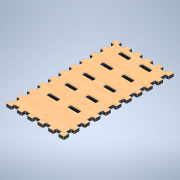
# Autodesk Inventor part: plate_top_middle
Saved by Autodesk Inventor 2021 (Build 250183000, 183)
## iProperties
Created: 2021-03-07
Part Number: plate_top_middle
Material: Holz (Kirsche)
Document SubType Name: Modeling
Designer: Tilman
Density: 0.63 g/cm^3
Appearance: Glänzend - Schwarz
Author: Tilman
Autodesk Inventor part; units mm, degrees
ref_plane "YZ Plane" through (0, 0, 0) normal (1, 0, 0) x (0, 1, 0)
ref_plane "XZ Plane" through (0, 0, 0) normal (0, 1, 0) x (-1, 0, 0)
ref_plane "XY Plane" through (0, 0, 0) normal (0, 0, 1) x (1, 0, 0)
sketch "Skizze1" plane through (0, 0, 0) normal (0, 1, 0) x (-1, 0, 0)
  line L0 (-12.5, -26) -> (-22.5, -26)
  line L1 (-22.5, -26) -> (-22.5, -29)
  line L2 (-22.5, -29) -> (-12.5, -29)
  line L3 (-12.5, -29) -> (-12.5, -26)
  line L4 (-32.5, -26) -> (-42.5, -26)
  line L5 (-42.5, -26) -> (-42.5, -29)
  line L6 (-42.5, -29) -> (-32.5, -29)
  line L7 (-32.5, -29) -> (-32.5, -26)
  line L8 (-12.5, -43) -> (-22.5, -43)
  line L9 (-22.5, -43) -> (-22.5, -46)
  line L10 (-22.5, -46) -> (-12.5, -46)
  line L11 (-12.5, -46) -> (-12.5, -43)
  line L12 (-32.5, -43) -> (-42.5, -43)
  line L13 (-42.5, -43) -> (-42.5, -46)
  line L14 (-42.5, -46) -> (-32.5, -46)
  line L15 (-32.5, -46) -> (-32.5, -43)
  line L16 (-12.5, -60) -> (-22.5, -60)
  line L17 (-22.5, -60) -> (-22.5, -63)
  line L18 (-22.5, -63) -> (-12.5, -63)
  line L19 (-12.5, -63) -> (-12.5, -60)
  line L20 (-32.5, -60) -> (-42.5, -60)
  line L21 (-42.5, -60) -> (-42.5, -63)
  line L22 (-42.5, -63) -> (-32.5, -63)
  line L23 (-32.5, -63) -> (-32.5, -60)
  line L24 (-12.5, -77) -> (-22.5, -77)
  line L25 (-22.5, -77) -> (-22.5, -80)
  line L26 (-22.5, -80) -> (-12.5, -80)
  line L27 (-12.5, -80) -> (-12.5, -77)
  line L28 (-32.5, -77) -> (-42.5, -77)
  line L29 (-42.5, -77) -> (-42.5, -80)
  line L30 (-42.5, -80) -> (-32.5, -80)
  line L31 (-32.5, -80) -> (-32.5, -77)
  line L32 (-12.5, -94) -> (-22.5, -94)
  line L33 (-22.5, -94) -> (-22.5, -97)
  line L34 (-22.5, -97) -> (-12.5, -97)
  line L35 (-12.5, -97) -> (-12.5, -94)
  line L36 (-32.5, -94) -> (-42.5, -94)
  line L37 (-42.5, -94) -> (-42.5, -97)
  line L38 (-42.5, -97) -> (-32.5, -97)
  line L39 (-32.5, -97) -> (-32.5, -94)
  line L40 (0, 0) -> (-5, 0)
  line L41 (-5, 0) -> (-5, -3)
  line L42 (-5, -3) -> (-10, -3)
  line L43 (-10, -3) -> (-10, 0)
  line L44 (-20, -3) -> (-20, 0)
  line L45 (-15, -3) -> (-20, -3)
  line L46 (-15, 0) -> (-15, -3)
  line L47 (-10, 0) -> (-15, 0)
  line L48 (-30, -3) -> (-30, 0)
  line L49 (-25, -3) -> (-30, -3)
  line L50 (-25, 0) -> (-25, -3)
  line L51 (-20, 0) -> (-25, 0)
  line L52 (-40, -3) -> (-40, 0)
  line L53 (-35, -3) -> (-40, -3)
  line L54 (-35, 0) -> (-35, -3)
  line L55 (-30, 0) -> (-35, 0)
  line L56 (-50, -3) -> (-50, 0)
  line L57 (-45, -3) -> (-50, -3)
  line L58 (-45, 0) -> (-45, -3)
  line L59 (-40, 0) -> (-45, 0)
  line L60 (-50, 0) -> (-55, 0)
  line L61 (-55, 0) -> (-55, -5)
  line L62 (-55, -5) -> (-52, -5)
  line L63 (-52, -5) -> (-52, -10)
  line L64 (-52, -10) -> (-55, -10)
  line L65 (-52, -15) -> (-52, -20)
  line L66 (-55, -10) -> (-55, -15)
  line L67 (-55, -15) -> (-52, -15)
  line L68 (-52, -20) -> (-55, -20)
  line L69 (-52, -25) -> (-52, -30)
  line L70 (-55, -20) -> (-55, -25)
  line L71 (-55, -25) -> (-52, -25)
  line L72 (-52, -30) -> (-55, -30)
  line L73 (-52, -35) -> (-52, -40)
  line L74 (-55, -30) -> (-55, -35)
  line L75 (-55, -35) -> (-52, -35)
  line L76 (-52, -40) -> (-55, -40)
  line L77 (-52, -45) -> (-52, -50)
  line L78 (-55, -40) -> (-55, -45)
  line L79 (-55, -45) -> (-52, -45)
  line L80 (-52, -50) -> (-55, -50)
  line L81 (-52, -55) -> (-52, -60)
  line L82 (-55, -50) -> (-55, -55)
  line L83 (-55, -55) -> (-52, -55)
  line L84 (-52, -60) -> (-55, -60)
  line L85 (-52, -65) -> (-52, -70)
  line L86 (-55, -60) -> (-55, -65)
  line L87 (-55, -65) -> (-52, -65)
  line L88 (-52, -70) -> (-55, -70)
  line L89 (-52, -75) -> (-52, -80)
  line L90 (-55, -70) -> (-55, -75)
  line L91 (-55, -75) -> (-52, -75)
  line L92 (-52, -80) -> (-55, -80)
  line L93 (-22.5, -61.5) -> (-32.5, -61.5) construction
  line L94 (-27.5, -105) -> (-27.5, 0) construction
  line L95 (-55, -80) -> (-55, -85)
  line L96 (-55, -105) -> (-50, -105)
  line L97 (-50, -105) -> (-50, -102)
  line L98 (-50, -102) -> (-45, -102)
  line L99 (-45, -102) -> (-45, -105)
  line L100 (-40, -102) -> (-35, -102)
  line L101 (-35, -102) -> (-35, -105)
  line L102 (-40, -105) -> (-40, -102)
  line L103 (-45, -105) -> (-40, -105)
  line L104 (-30, -102) -> (-25, -102)
  line L105 (-25, -102) -> (-25, -105)
  line L106 (-30, -105) -> (-30, -102)
  line L107 (-35, -105) -> (-30, -105)
  line L108 (-20, -102) -> (-15, -102)
  line L109 (-15, -102) -> (-15, -105)
  line L110 (-20, -105) -> (-20, -102)
  line L111 (-25, -105) -> (-20, -105)
  line L112 (-10, -102) -> (-5, -102)
  line L113 (-5, -102) -> (-5, -105)
  line L114 (-10, -105) -> (-10, -102)
  line L115 (-15, -105) -> (-10, -105)
  line L116 (-5, -105) -> (0, -105)
  line L117 (0, -105) -> (0, -100)
  line L118 (0, -100) -> (-3, -100)
  line L119 (-3, -100) -> (-3, -95)
  line L120 (-3, -95) -> (0, -95)
  line L121 (-3, -90) -> (-3, -85)
  line L122 (-3, -85) -> (0, -85)
  line L123 (0, -90) -> (-3, -90)
  line L124 (0, -95) -> (0, -90)
  line L125 (-3, -80) -> (-3, -75)
  line L126 (-3, -75) -> (0, -75)
  line L127 (0, -80) -> (-3, -80)
  line L128 (0, -85) -> (0, -80)
  line L129 (-3, -70) -> (-3, -65)
  line L130 (-3, -65) -> (0, -65)
  line L131 (0, -70) -> (-3, -70)
  line L132 (0, -75) -> (0, -70)
  line L133 (-3, -60) -> (-3, -55)
  line L134 (-3, -55) -> (0, -55)
  line L135 (0, -60) -> (-3, -60)
  line L136 (0, -65) -> (0, -60)
  line L137 (-3, -50) -> (-3, -45)
  line L138 (-3, -45) -> (0, -45)
  line L139 (0, -50) -> (-3, -50)
  line L140 (0, -55) -> (0, -50)
  line L141 (-3, -40) -> (-3, -35)
  line L142 (-3, -35) -> (0, -35)
  line L143 (0, -40) -> (-3, -40)
  line L144 (0, -45) -> (0, -40)
  line L145 (-3, -30) -> (-3, -25)
  line L146 (-3, -25) -> (0, -25)
  line L147 (0, -30) -> (-3, -30)
  line L148 (0, -35) -> (0, -30)
  line L149 (-52, -85) -> (-52, -90)
  line L150 (-55, -80) -> (-55, -85)
  line L151 (-55, -85) -> (-52, -85)
  line L152 (-52, -90) -> (-55, -90)
  line L153 (-3, -20) -> (-3, -15)
  line L154 (-3, -15) -> (0, -15)
  line L155 (0, -20) -> (-3, -20)
  line L156 (0, -25) -> (0, -20)
  line L157 (-52, -95) -> (-52, -100)
  line L158 (-55, -90) -> (-55, -95)
  line L159 (-55, -95) -> (-52, -95)
  line L160 (-52, -100) -> (-55, -100)
  line L161 (-3, -10) -> (-3, -5)
  line L162 (-3, -5) -> (0, -5)
  line L163 (0, -10) -> (-3, -10)
  line L164 (0, -15) -> (0, -10)
  line L165 (-55, -100) -> (-55, -105)
  line L166 (0, -5) -> (0, 0)
  line L167 (-3, -10) -> (-52, -10) construction
  point P0 (-27.5, -61.5)
  point P1 (-27.5, -10)
  dimension "d0" = 10
  dimension "d1" = 3
  dimension "d4" = 20
  dimension "d7" = 17
  dimension "d10" = 5
  dimension "d11" = 3
  dimension "d15" = 10
  dimension "d22" = 10
  dimension "d31" = 10
  dimension "d38" = 10
  dimension "d45" = 5
  constraints: 336 end point, 31 point on line, 15 perpendicular, 14 equal length, 8 horizontal, 6 collinear, 6 vertical, 4 midpoint, 2 horizontal alignment, 2 parallel, 1 coincident, 1 vertical alignment, 300 other
  measures "d0" distance of L2.end L1.end
  measures "d1" distance of L1.end L0.end
  measures "d4" distance of L0.start L4.start
  measures "d7" distance of L0.start L8.start
  measures "d10" distance of L40.start L40.end
  measures "d11" distance of L40.end L41.end
  measures "d15" distance of L42.end L44.start
  measures "d22" distance of L63.end L65.end
  measures "d31" distance of L98.end L100.end
  measures "d38" distance of L118.end L121.start
  measures "d45" distance between parallel lines of L108 L34
extrude "Extrusion1" add sketch "Skizze1" along normal blind 3
